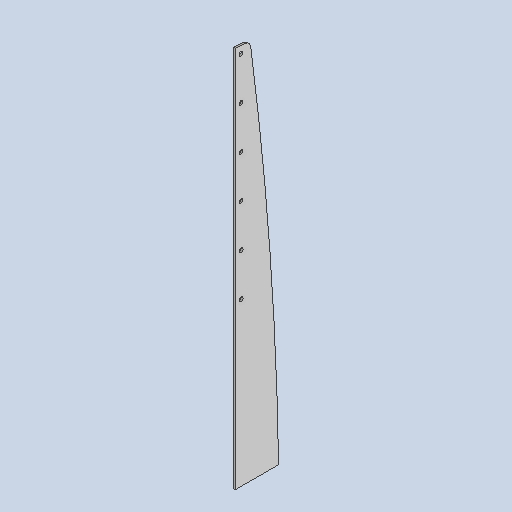
# Autodesk Inventor part: MSC 083 top support gills
Saved by Autodesk Inventor 2025 (Build 290162010, 162A)
## iProperties
Created: 2024-08-30
Part Number: MSC 083 top support gills
Material: Stainless Steel
Document SubType Name: Sheet Metal
Designer: pokla
Density: 8 g/cm^3
Sheet Metal Rule: AISI304 3mm Die 32
Appearance: Default
Stock Number: МОО 083 верхняя консоль жабры
Author: pokla
Autodesk Inventor part; units mm, degrees
ref_plane "YZ Plane" through (0, 0, 0) normal (1, 0, 0) x (0, 1, 0)
ref_plane "XZ Plane" through (0, 0, 0) normal (0, 1, 0) x (-1, 0, 0)
ref_plane "XY Plane" through (0, 0, 0) normal (0, 0, 1) x (1, 0, 0)
sketch "Sketch1" plane through (0, 0, 0) normal (1, 0, 0) x (0, 1, 0)
  line L0 (25, 748.8121) -> (0, 748.8121)
  line L1 (0, 748.8121) -> (0, -748.8121)
  line L2 (0, -748.8121) -> (25, -748.8121)
  arc A0 (25, -748.8121) -> (25, 748.8121) centre (-5575.159, 0) ccw
  line L3 (0, 748.8121) -> (25.2835, 746.689)
  line L4 (0, -748.8121) -> (25.2835, -746.689)
  line L5 (0, 97) -> (74.0083, 97)
  point P0 (0, 0)
  point P1 (0, 0)
  dimension "d2" = 25
  dimension "d3" = 5650
  dimension "d7" = 85.2
  dimension "d8" = 85.2
  dimension "d33" = 97
  dimension "d34" = 651.812
  measures "d2" distance of L0.start L0.end
  measures "d3" radius of A0
  measures "d7" angle of L1 L3
  measures "d8" angle of L1 L4
  measures "d33" distance of point (0, 0) L5.start
  measures "d34" distance from line of L0.end L5
extrude "Plate1" add sketch "Sketch1" against normal blind 3.048 contours L3 A0 L5 L1
fillet "Corner Round3" radius 10 1 edges at (-1.524, 25.2835, 746.689)
sketch "Sketch4" plane through (0, 0, 0) normal (1, 0, 0) x (0, 0, -1)
  circle A0 centre (-735.8121, 10) radius 3.5
  line L0 (-748.8121, 0) -> (-97, 0) projected
  point P0 (0, 0)
  dimension "d23" = 7
  dimension "d25" = 10
  dimension "d32" = 13
  constraints: 1 centre point
  measures "d23" diameter of A0
  measures "d25" distance from line of L0 A0.centre
  measures "d32" horizontal distance of A0.centre L0.start
extrude "Extrusion1" cut sketch "Sketch4" against normal through all
pattern_linear "Rectangular Pattern2" count 6 spacing 72.5 along (0, 0, -1) of "Extrusion1"
equation "\"BendReliefWidth\" = Thickness"
equation "\"BendReliefDepth\" = 0.5 * Thickness"
equation "\"CornerReliefSize\" = 4 * Thickness"
equation "\"MinimumRemnant\" = 2 * Thickness"
equation "\"TransitionRadius\" = BendRadius"
equation "\"JacobiRadiusSize\" = BendRadius"
equation "\"GapSize\" = Thickness"
equation "\"BendRadius\" = Thickness"
body "Solid1"
